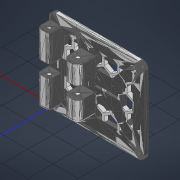
# Autodesk Inventor part: voron_2.4_7in_pi_base
Saved by Autodesk Inventor 2022.2 (Build 262287010, 287A)
## iProperties
Created: 2022-03-18
Part Number: voron_2.4_7in_pi_base
Material: Generisch
Document SubType Name: Modeling
Designer: sleib
Density: 1 g/cm^3
Appearance: Vorgabe
Author: sleib
Autodesk Inventor part; units mm, degrees
ref_plane "YZ Plane" through (0, 0, 0) normal (1, 0, 0) x (0, 1, 0)
ref_plane "XZ Plane" through (0, 0, 0) normal (0, 1, 0) x (-1, 0, 0)
ref_plane "XY Plane" through (0, 0, 0) normal (0, 0, 1) x (1, 0, 0)
sketch "Skizze1" plane through (21.42, 0, 3) normal (0, 0, -1) x (-1, 0, 0)
  line L0 (-53.75, 67) -> (21.25, 67)
  line L1 (21.25, 67) -> (21.25, 0)
  line L2 (21.25, 0) -> (-53.75, 0)
  line L3 (-53.75, 0) -> (-53.75, 67)
  circle A0 centre (-49.25, 62.5) radius 2
  circle A1 centre (-0.25, 62.5) radius 2
  circle A2 centre (-49.25, 4.5) radius 2
  circle A3 centre (-0.25, 4.5) radius 2
  line L4 (-28.4468, 44.8124) -> (-37, 54.875)
  line L5 (-37, 54.875) -> (-16.25, 54.875)
  line L6 (-16.25, 54.875) -> (-16.25, 44.875)
  line L7 (-16.25, 44.875) -> (-28.5, 44.875)
  line L8 (-37, 12.125) -> (-28.5, 22.125)
  line L9 (-28.5, 22.125) -> (-16.25, 22.125)
  line L10 (-16.25, 22.125) -> (-16.25, 12.125)
  line L11 (-16.25, 12.125) -> (-37, 12.125)
  line L12 (-34.75, 34.5) -> (-14.75, 34.5)
  line L13 (-14.75, 34.5) -> (-14.75, 32.5)
  line L14 (-14.75, 32.5) -> (-34.75, 32.5)
  line L15 (-34.75, 32.5) -> (-34.75, 34.5)
  line L16 (-1.75, 55.25) -> (9.5, 55.25)
  line L17 (9.5, 55.25) -> (9.5, 39.25)
  line L18 (9.5, 39.25) -> (-1.75, 39.25)
  line L19 (-1.75, 39.25) -> (-1.75, 55.25)
  line L20 (-1.75, 27.75) -> (9.5, 27.75)
  line L21 (9.5, 27.75) -> (9.5, 11.75)
  line L22 (9.5, 11.75) -> (-1.75, 11.75)
  line L23 (-1.75, 11.75) -> (-1.75, 27.75)
  line L24 (-44.75, 17) -> (-44.75, 50)
  line L25 (-44.75, 50) -> (-36.75, 40.5)
  line L26 (-36.75, 40.5) -> (-36.75, 26.5)
  line L27 (-36.75, 26.5) -> (-44.75, 17)
  arc A4 (16.75, 0) -> (21.25, 4.5) centre (16.75, 4.5) ccw
  arc A5 (21.25, 62.5) -> (16.75, 67) centre (16.75, 62.5) ccw
  arc A6 (-49.25, 67) -> (-53.75, 62.5) centre (-49.25, 62.5) ccw
  arc A7 (-53.75, 4.5) -> (-49.25, 0) centre (-49.25, 4.5) ccw
  line L28 (-53.75, 33.5) -> (21.25, 33.5) construction
  line L29 (21.25, 60) -> (12, 60)
  line L30 (12, 60) -> (12, 38.5)
  line L31 (12, 38.5) -> (21.25, 38.5)
  line L32 (21.25, 38.5) -> (21.25, 60)
  line L33 (21.25, 28.5) -> (12, 28.5)
  line L34 (12, 28.5) -> (12, 7)
  line L35 (12, 7) -> (21.25, 7)
  line L36 (21.25, 7) -> (21.25, 28.5)
  line L37 (-3.75, 28.5) -> (-14.75, 28.5)
  line L38 (-14.75, 28.5) -> (-14.75, 13.75)
  line L39 (-14.75, 13.75) -> (-3.75, 13.75)
  line L40 (-3.75, 13.75) -> (-3.75, 28.5)
  line L41 (-14.75, 38.5) -> (-3.75, 38.5)
  line L42 (-3.75, 38.5) -> (-3.75, 53.25)
  line L43 (-3.75, 53.25) -> (-14.75, 53.25)
  line L44 (-14.75, 53.25) -> (-14.75, 38.5)
  circle A8 centre (-0.25, 4.5) radius 3.25
  circle A9 centre (-0.25, 62.5) radius 3.25
  circle A10 centre (-49.25, 62.5) radius 3.25
  circle A11 centre (-49.25, 4.5) radius 3.25
  point P0 (0, 0)
  dimension "d0" = 67
  dimension "d1" = 75
  dimension "d2" = 9
  dimension "d3" = 8
  dimension "d4" = 33
  dimension "d5" = 14
  dimension "d7" = 4
  dimension "d8" = 4.5
  dimension "d9" = 2
  dimension "d10" = 20
  dimension "d11" = 19
  dimension "d12" = 20.75
  dimension "d13" = 12.25
  dimension "d14" = 10
  dimension "d15" = 16
  dimension "d16" = 11.25
  dimension "d17" = 11.5
  dimension "d18" = 22.75
  dimension "d19" = 11.75
  dimension "d20" = 21.5
  dimension "d21" = 21.25
  dimension "d22" = 37.5
  dimension "d23" = 9.25
  dimension "d24" = 10
  dimension "d25" = 14.75
  dimension "d26" = 21.5
  dimension "d27" = 11
  dimension "d28" = 25
  dimension "d114" = 6.5
  constraints: 90 end point, 19 parallel, 17 point on line, 12 centre point, 11 perpendicular, 9 horizontal, 8 equal radius, 8 point on circle, 8 tangent, 6 coincident, 2 collinear, 2 horizontal alignment, 2 midpoint, 2 symmetric about line, 2 vertical, 10 other
  measures "d0" distance between parallel lines of L2 L0
  measures "d1" distance between parallel lines of L1 L3
  measures "d2" distance between parallel lines of L3 L24
  measures "d3" distance between parallel lines of L26 L24
  measures "d4" distance of L24.start L24.end
  measures "d5" distance of L25.end L26.end
  measures "d7" diameter of A0
  measures "d8" radius of A6
  measures "d9" distance between parallel lines of L14 L12
  measures "d10" distance between parallel lines of L13 L15
  measures "d11" distance between parallel lines of L15 L3
  measures "d12" distance of L4.end L5.end
  measures "d13" distance of L6.end L7.end
  measures "d14" distance of L5.end L6.end
  measures "d15" distance between parallel lines of L18 L16
  measures "d16" distance between parallel lines of L17 L19
  measures "d17" distance between parallel lines of L20 L18
  measures "d18" distance between parallel lines of L9 L7
  measures "d19" distance between parallel lines of L1 L17
  measures "d20" distance from line of L1 A1.centre
  measures "d21" distance from line of L1 point (0, 0)
  measures "d22" distance between parallel lines of L6 L1
  measures "d23" distance between parallel lines of L30 L1
  measures "d24" distance between parallel lines of L33 L31
  measures "d25" distance of L41.end L42.end
  measures "d26" distance between parallel lines of L31 L29
  measures "d27" distance between parallel lines of L42 L44
  measures "d28" distance between parallel lines of L1 L42
  measures "d114" diameter of A10
extrude "Extrusion1" add sketch "Skizze1" along normal blind 3 contours L0 A5 L1 L29 L30 L31 L33 L34 L35 A4 L2 A7 L3 A6 | L1 L31 L30 L29 | L1 L35 L34 L33 | L4 L5 L6 L7 | L8 L9 L10 L11 | L12 L13 L14 L15 | L16 L17 L18 L19 | L20 L21 L22 L23 | L24 L25 L26 L27 | L40 L39 L38 L37 | L44 L43 L42 L41 | A8 | A9 | A10 | A11
sketch "Skizze3" plane through (21.42, 0, 3) normal (0, 0, 1) x (-1, 0, 0)
  line L0 (21.25, -4.5) -> (21.25, -62.5) projected
  arc A0 (16.75, -67) -> (21.25, -62.5) centre (16.75, -62.5) ccw projected
  line L1 (16.75, -67) -> (-49.25, -67) projected
  arc A1 (-53.75, -62.5) -> (-49.25, -67) centre (-49.25, -62.5) ccw projected
  line L2 (-53.75, -62.5) -> (-53.75, -4.5) projected
  arc A2 (-49.25, 0) -> (-53.75, -4.5) centre (-49.25, -4.5) ccw projected
  line L3 (-49.25, 0) -> (16.75, 0) projected
  arc A3 (21.25, -4.5) -> (16.75, 0) centre (16.75, -4.5) ccw projected
  circle A4 centre (-0.25, -62.5) radius 2 projected
  circle A5 centre (-0.25, -4.5) radius 2 projected
  circle A6 centre (-49.25, -4.5) radius 2 projected
  circle A7 centre (-49.25, -62.5) radius 2 projected
  line L4 (3.75, -16.3868) -> (3.75, -10.6132)
  line L5 (3.75, -10.6132) -> (8.75, -7.7265)
  line L6 (8.75, -7.7265) -> (13.75, -10.6132)
  line L7 (13.75, -10.6132) -> (13.75, -16.3868)
  line L8 (13.75, -16.3868) -> (8.75, -19.2735)
  line L9 (8.75, -19.2735) -> (3.75, -16.3868)
  line L10 (14.75, -29.2735) -> (9.75, -26.3868)
  line L11 (9.75, -26.3868) -> (9.75, -20.6132)
  line L12 (9.75, -20.6132) -> (14.75, -17.7265)
  line L13 (14.75, -17.7265) -> (19.75, -20.6132)
  line L14 (19.75, -20.6132) -> (19.75, -26.3868)
  line L15 (19.75, -26.3868) -> (14.75, -29.2735)
  line L16 (21.25, -62.5) -> (21.25, -4.5) projected
  line L17 (21.25, -33.5) -> (-53.75, -33.5) construction
  line L18 (-53.75, -62.5) -> (-53.75, -4.5) projected
  line L19 (13.75, -30.6132) -> (13.75, -36.3868)
  line L20 (8.75, -27.7265) -> (13.75, -30.6132)
  line L21 (3.75, -30.6132) -> (8.75, -27.7265)
  line L22 (13.75, -36.3868) -> (8.75, -39.2735)
  line L23 (3.75, -36.3868) -> (3.75, -30.6132)
  line L24 (8.75, -39.2735) -> (3.75, -36.3868)
  line L25 (13.75, -50.6132) -> (13.75, -56.3868)
  line L26 (8.75, -47.7265) -> (13.75, -50.6132)
  line L27 (3.75, -50.6132) -> (8.75, -47.7265)
  line L28 (13.75, -56.3868) -> (8.75, -59.2735)
  line L29 (3.75, -56.3868) -> (3.75, -50.6132)
  line L30 (8.75, -59.2735) -> (3.75, -56.3868)
  line L31 (1.75, -10.6132) -> (1.75, -16.3868)
  line L32 (-3.25, -7.7265) -> (1.75, -10.6132)
  line L33 (-8.25, -10.6132) -> (-3.25, -7.7265)
  line L34 (1.75, -16.3868) -> (-3.25, -19.2735)
  line L35 (-8.25, -16.3868) -> (-8.25, -10.6132)
  line L36 (-3.25, -19.2735) -> (-8.25, -16.3868)
  line L37 (1.75, -30.6132) -> (1.75, -36.3868)
  line L38 (-3.25, -27.7265) -> (1.75, -30.6132)
  line L39 (-8.25, -30.6132) -> (-3.25, -27.7265)
  line L40 (1.75, -36.3868) -> (-3.25, -39.2735)
  line L41 (-8.25, -36.3868) -> (-8.25, -30.6132)
  line L42 (-3.25, -39.2735) -> (-8.25, -36.3868)
  line L43 (1.75, -50.6132) -> (1.75, -56.3868)
  line L44 (-3.25, -47.7265) -> (1.75, -50.6132)
  line L45 (-8.25, -50.6132) -> (-3.25, -47.7265)
  line L46 (1.75, -56.3868) -> (-3.25, -59.2735)
  line L47 (-8.25, -56.3868) -> (-8.25, -50.6132)
  line L48 (-3.25, -59.2735) -> (-8.25, -56.3868)
  line L49 (-10.25, -10.6132) -> (-10.25, -16.3868)
  line L50 (-15.25, -7.7265) -> (-10.25, -10.6132)
  line L51 (-20.25, -10.6132) -> (-15.25, -7.7265)
  line L52 (-10.25, -16.3868) -> (-15.25, -19.2735)
  line L53 (-20.25, -16.3868) -> (-20.25, -10.6132)
  line L54 (-15.25, -19.2735) -> (-20.25, -16.3868)
  line L55 (-10.25, -30.6132) -> (-10.25, -36.3868)
  line L56 (-15.25, -27.7265) -> (-10.25, -30.6132)
  line L57 (-20.25, -30.6132) -> (-15.25, -27.7265)
  line L58 (-10.25, -36.3868) -> (-15.25, -39.2735)
  line L59 (-20.25, -36.3868) -> (-20.25, -30.6132)
  line L60 (-15.25, -39.2735) -> (-20.25, -36.3868)
  line L61 (-10.25, -50.6132) -> (-10.25, -56.3868)
  line L62 (-15.25, -47.7265) -> (-10.25, -50.6132)
  line L63 (-20.25, -50.6132) -> (-15.25, -47.7265)
  line L64 (-10.25, -56.3868) -> (-15.25, -59.2735)
  line L65 (-20.25, -56.3868) -> (-20.25, -50.6132)
  line L66 (-15.25, -59.2735) -> (-20.25, -56.3868)
  line L67 (-22.25, -10.6132) -> (-22.25, -16.3868)
  line L68 (-27.25, -7.7265) -> (-22.25, -10.6132)
  line L69 (-32.25, -10.6132) -> (-27.25, -7.7265)
  line L70 (-22.25, -16.3868) -> (-27.25, -19.2735)
  line L71 (-32.25, -16.3868) -> (-32.25, -10.6132)
  line L72 (-27.25, -19.2735) -> (-32.25, -16.3868)
  line L73 (-22.25, -30.6132) -> (-22.25, -36.3868)
  line L74 (-27.25, -27.7265) -> (-22.25, -30.6132)
  line L75 (-32.25, -30.6132) -> (-27.25, -27.7265)
  line L76 (-22.25, -36.3868) -> (-27.25, -39.2735)
  line L77 (-32.25, -36.3868) -> (-32.25, -30.6132)
  line L78 (-27.25, -39.2735) -> (-32.25, -36.3868)
  line L79 (-22.25, -50.6132) -> (-22.25, -56.3868)
  line L80 (-27.25, -47.7265) -> (-22.25, -50.6132)
  line L81 (-32.25, -50.6132) -> (-27.25, -47.7265)
  line L82 (-22.25, -56.3868) -> (-27.25, -59.2735)
  line L83 (-32.25, -56.3868) -> (-32.25, -50.6132)
  line L84 (-27.25, -59.2735) -> (-32.25, -56.3868)
  line L85 (-34.25, -10.6132) -> (-34.25, -16.3868)
  line L86 (-39.25, -7.7265) -> (-34.25, -10.6132)
  line L87 (-44.25, -10.6132) -> (-39.25, -7.7265)
  line L88 (-34.25, -16.3868) -> (-39.25, -19.2735)
  line L89 (-44.25, -16.3868) -> (-44.25, -10.6132)
  line L90 (-39.25, -19.2735) -> (-44.25, -16.3868)
  line L91 (-34.25, -30.6132) -> (-34.25, -36.3868)
  line L92 (-39.25, -27.7265) -> (-34.25, -30.6132)
  line L93 (-44.25, -30.6132) -> (-39.25, -27.7265)
  line L94 (-34.25, -36.3868) -> (-39.25, -39.2735)
  line L95 (-44.25, -36.3868) -> (-44.25, -30.6132)
  line L96 (-39.25, -39.2735) -> (-44.25, -36.3868)
  line L97 (-34.25, -50.6132) -> (-34.25, -56.3868)
  line L98 (-39.25, -47.7265) -> (-34.25, -50.6132)
  line L99 (-44.25, -50.6132) -> (-39.25, -47.7265)
  line L100 (-34.25, -56.3868) -> (-39.25, -59.2735)
  line L101 (-44.25, -56.3868) -> (-44.25, -50.6132)
  line L102 (-39.25, -59.2735) -> (-44.25, -56.3868)
  line L103 (9.75, -40.6132) -> (14.75, -37.7265)
  line L104 (14.75, -49.2735) -> (9.75, -46.3868)
  line L105 (14.75, -37.7265) -> (19.75, -40.6132)
  line L106 (9.75, -46.3868) -> (9.75, -40.6132)
  line L107 (19.75, -40.6132) -> (19.75, -46.3868)
  line L108 (19.75, -46.3868) -> (14.75, -49.2735)
  line L109 (-2.25, -20.6132) -> (2.75, -17.7265)
  line L110 (2.75, -29.2735) -> (-2.25, -26.3868)
  line L111 (2.75, -17.7265) -> (7.75, -20.6132)
  line L112 (-2.25, -26.3868) -> (-2.25, -20.6132)
  line L113 (7.75, -20.6132) -> (7.75, -26.3868)
  line L114 (7.75, -26.3868) -> (2.75, -29.2735)
  line L115 (-2.25, -40.6132) -> (2.75, -37.7265)
  line L116 (2.75, -49.2735) -> (-2.25, -46.3868)
  line L117 (2.75, -37.7265) -> (7.75, -40.6132)
  line L118 (-2.25, -46.3868) -> (-2.25, -40.6132)
  line L119 (7.75, -40.6132) -> (7.75, -46.3868)
  line L120 (7.75, -46.3868) -> (2.75, -49.2735)
  line L121 (-14.25, -20.6132) -> (-9.25, -17.7265)
  line L122 (-9.25, -29.2735) -> (-14.25, -26.3868)
  line L123 (-9.25, -17.7265) -> (-4.25, -20.6132)
  line L124 (-14.25, -26.3868) -> (-14.25, -20.6132)
  line L125 (-4.25, -20.6132) -> (-4.25, -26.3868)
  line L126 (-4.25, -26.3868) -> (-9.25, -29.2735)
  line L127 (-14.25, -40.6132) -> (-9.25, -37.7265)
  line L128 (-9.25, -49.2735) -> (-14.25, -46.3868)
  line L129 (-9.25, -37.7265) -> (-4.25, -40.6132)
  line L130 (-14.25, -46.3868) -> (-14.25, -40.6132)
  line L131 (-4.25, -40.6132) -> (-4.25, -46.3868)
  line L132 (-4.25, -46.3868) -> (-9.25, -49.2735)
  line L133 (-26.25, -20.6132) -> (-21.25, -17.7265)
  line L134 (-21.25, -29.2735) -> (-26.25, -26.3868)
  line L135 (-21.25, -17.7265) -> (-16.25, -20.6132)
  line L136 (-26.25, -26.3868) -> (-26.25, -20.6132)
  line L137 (-16.25, -20.6132) -> (-16.25, -26.3868)
  line L138 (-16.25, -26.3868) -> (-21.25, -29.2735)
  line L139 (-26.25, -40.6132) -> (-21.25, -37.7265)
  line L140 (-21.25, -49.2735) -> (-26.25, -46.3868)
  line L141 (-21.25, -37.7265) -> (-16.25, -40.6132)
  line L142 (-26.25, -46.3868) -> (-26.25, -40.6132)
  line L143 (-16.25, -40.6132) -> (-16.25, -46.3868)
  line L144 (-16.25, -46.3868) -> (-21.25, -49.2735)
  line L145 (-38.25, -20.6132) -> (-33.25, -17.7265)
  line L146 (-33.25, -29.2735) -> (-38.25, -26.3868)
  line L147 (-33.25, -17.7265) -> (-28.25, -20.6132)
  line L148 (-38.25, -26.3868) -> (-38.25, -20.6132)
  line L149 (-28.25, -20.6132) -> (-28.25, -26.3868)
  line L150 (-28.25, -26.3868) -> (-33.25, -29.2735)
  line L151 (-38.25, -40.6132) -> (-33.25, -37.7265)
  line L152 (-33.25, -49.2735) -> (-38.25, -46.3868)
  line L153 (-33.25, -37.7265) -> (-28.25, -40.6132)
  line L154 (-38.25, -46.3868) -> (-38.25, -40.6132)
  line L155 (-28.25, -40.6132) -> (-28.25, -46.3868)
  line L156 (-28.25, -46.3868) -> (-33.25, -49.2735)
  line L157 (-50.25, -20.6132) -> (-45.25, -17.7265)
  line L158 (-45.25, -29.2735) -> (-50.25, -26.3868)
  line L159 (-45.25, -17.7265) -> (-40.25, -20.6132)
  line L160 (-50.25, -26.3868) -> (-50.25, -20.6132)
  line L161 (-40.25, -20.6132) -> (-40.25, -26.3868)
  line L162 (-40.25, -26.3868) -> (-45.25, -29.2735)
  line L163 (-50.25, -40.6132) -> (-45.25, -37.7265)
  line L164 (-45.25, -49.2735) -> (-50.25, -46.3868)
  line L165 (-45.25, -37.7265) -> (-40.25, -40.6132)
  line L166 (-50.25, -46.3868) -> (-50.25, -40.6132)
  line L167 (-40.25, -40.6132) -> (-40.25, -46.3868)
  line L168 (-40.25, -46.3868) -> (-45.25, -49.2735)
  point P0 (21.42, 0)
  point P1 (8.75, -13.5)
  point P2 (14.75, -23.5)
  point P3 (21.25, 38.5)
  point P4 (21.25, 28.5)
  point P5 (8.75, -33.5)
  point P6 (8.75, -53.5)
  point P7 (-3.25, -13.5)
  point P8 (-3.25, -33.5)
  point P9 (-3.25, -53.5)
  point P10 (-15.25, -13.5)
  point P11 (-15.25, -33.5)
  point P12 (-15.25, -53.5)
  point P13 (-27.25, -13.5)
  point P14 (-27.25, -33.5)
  point P15 (-27.25, -53.5)
  point P16 (-39.25, -13.5)
  point P17 (-39.25, -33.5)
  point P18 (-39.25, -53.5)
  point P19 (8.75, -39.2735)
  point P20 (14.75, -43.5)
  point P21 (8.75, -47.7265)
  point P22 (2.75, -23.5)
  point P23 (-3.25, -39.2735)
  point P24 (2.75, -43.5)
  point P25 (-3.25, -47.7265)
  point P26 (-9.25, -23.5)
  point P27 (-15.25, -39.2735)
  point P28 (-9.25, -43.5)
  point P29 (-15.25, -47.7265)
  point P30 (-21.25, -23.5)
  point P31 (-21.25, -43.5)
  point P32 (-27.25, -47.7265)
  point P33 (-33.25, -23.5)
  point P34 (-33.25, -43.5)
  point P35 (-51.25, -19.2735)
  point P36 (-45.25, -23.5)
  point P37 (-51.25, -27.7265)
  point P38 (-51.25, -39.2735)
  point P39 (-45.25, -43.5)
  point P40 (-51.25, -47.7265)
  dimension "d72" = 10
  dimension "d74" = 10
  dimension "d82" = 20
  dimension "d85" = 12
  dimension "d90" = 20
  dimension "d93" = 12
  dimension "d96" = 10
  dimension "d97" = 1
  dimension "d98" = 7.5
  dimension "d99" = 9.5
  constraints: 326 end point, 4 vertical, 2 collinear, 2 horizontal, 2 midpoint, 1 point on line, 371 other
  measures "d72" distance between parallel lines of L4 L7
  measures "d74" distance between parallel lines of L11 L14
  measures "d82" distance of L6.end L19.start
  measures "d85" distance of L6.end L31.start
  measures "d90" distance of L13.start L103.end
  measures "d93" distance of L13.start L109.end
  measures "d96" vertical distance of point (14.75, -23.5) point (8.75, -13.5)
  measures "d97" distance from line of L11 point (8.75, -13.5)
  measures "d98" distance between parallel lines of L19 L0
  measures "d99" distance between parallel lines of L2 L95
extrude "Extrusion4" cut sketch "Skizze3" against normal through all contours L4 L5 L6 L7 L8 L9 | L19 L22 L24 L23 L21 L20 | L25 L28 L30 L29 L27 L26 | L31 L34 L36 L35 L33 L32 | L37 L40 L42 L41 L39 L38 | L43 L46 L48 L47 L45 L44 | L49 L52 L54 L53 L51 L50 | L55 L58 L60 L59 L57 L56 | L61 L64 L66 L65 L63 L62 | L67 L70 L72 L71 L69 L68 | L73 L76 L78 L77 L75 L74 | L79 L82 L84 L83 L81 L80 | L85 L88 L90 L89 L87 L86 | L91 L94 L96 L95 L93 L92 | L97 L100 L102 L101 L99 L98 | L109 L111 L113 L114 L110 L112 | L115 L117 L119 L120 L116 L118 | L133 L135 L137 L138 L134 L136 | L139 L141 L143 L144 L140 L142 | L145 L147 L149 L150 L146 L148 | L151 L153 L155 L156 L152 L154 | L157 L159 L161 L162 L158 L160 | L163 L165 L167 L168 L164 L166
extrude "Extrusion5" add sketch "Skizze1" along normal blind 3 and the other way blind 13.75 contours L40 L39 L38 L37 | L44 L43 L42 L41
extrude "Extrusion6" add sketch "Skizze1" along normal blind 3 and the other way blind 9.5 contours L1 L31 L30 L29 | L1 L35 L34 L33
extrude "Extrusion7" cut sketch "Skizze1" along normal blind 1 contours A8 | A9 | A10 | A11
fillet "Rundung1" radius 2.5 4 edges at (9.42, 49.25, 12.5) (0.17, 49.25, 12.5) (9.42, 17.75, 12.5) (0.17, 17.75, 12.5)
fillet "Rundung2" radius 4 4 edges at (25.17, 45.875, 16.75) (25.17, 21.125, 16.75) (36.17, 21.125, 16.75) (36.17, 45.875, 16.75)
